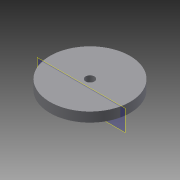
# Autodesk Inventor part: drive_wheel
Saved by Autodesk Inventor 2014 SP2 (Build 180246200, 246)
## iProperties
Created: 2015-11-29
Part Number: drive_wheel
Material: Generic
Document SubType Name: Modeling
Designer: schrluka
Mass: 11.8073 g
Surface Area: 48.793 cm^2
Volume: 11.8073 cm^3
Density: 1 g/cm^3
Appearance: Default
Author: schrluka
Autodesk Inventor part; units mm, degrees
ref_plane "YZ Plane" through (0, 0, 0) normal (1, 0, 0) x (0, 1, 0)
ref_plane "XY Plane" through (0, 0, 0) normal (0, 0, 1) x (1, 0, 0)
sketch "Sketch1" plane through (0, 0, 0) normal (0, 0, 1) x (1, 0, 0)
  circle A0 centre (71.5279, 0) radius 25.0279
  circle A1 centre (0, 0) radius 46.5 projected
  constraints: 1 centre point, 1 tangent
extrude "Extrusion1" add sketch "Sketch1" along normal mid plane 6 contours A0
sketch "Sketch2" plane through (71.5279, 0, -3) normal (0, 0, -1) x (-1, 0, 0)
  circle A0 centre (0, 0) radius 25.0279 projected
  circle A1 centre (0, 0) radius 5.5
  point P0 (71.5279, 0)
  dimension "d2" = 11
  constraints: 1 centre point, 1 coincident
  measures "d2" diameter of A1
extrude "Extrusion2" add sketch "Sketch2" along normal blind 6 contours A1
hole "Hole1" at (71.5279, 0, -9) direction (0, 0, 1) diameter 5.5 end through all
ref_plane "Work Plane1" through (71.5279, -5.5, -3) normal (0, 1, 0) x (-1, 0, 0)
sketch "Sketch3" plane through (71.5279, -5.5, -3) normal (0, 1, 0) x (-1, 0, 0)
  line L0 (-5.5, -6) -> (5.5, -6) projected
  line L1 (5.5, 0) -> (-5.5, 0) projected
  point P0 (71.5279, 3)
  point P1 (0.0146, -3)
  dimension "d14" = 3
  measures "d14" distance from line of point (0.015, -3) L0
hole "Hole2" at (71.5134, -5.5, -6) direction (0, 1, 0) diameter 3.5 end through all
body "Solid1"
